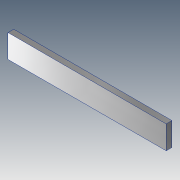
# Autodesk Inventor part: Y table support
Saved by Autodesk Inventor 2019 (Build 230136000, 136)
## iProperties
Created: 2018-10-20
Part Number: Y table support
Material: Aluminum 6061
Document SubType Name: Modeling
Designer: LillaHunden
Density: 2.7 g/cm^3
Appearance: Aluminum - Flat
Mass: 304.022 g
Surface Area: 289.886 cm^2
Volume: 112.601 cm^3
Author: LillaHunden
Autodesk Inventor part; units mm, degrees
ref_plane "YZ Plane" through (0, 0, 0) normal (1, 0, 0) x (0, 1, 0)
ref_plane "XZ Plane" through (0, 0, 0) normal (0, 1, 0) x (-1, 0, 0)
ref_plane "XY Plane" through (0, 0, 0) normal (0, 0, 1) x (1, 0, 0)
sketch "Sketch1" plane through (0, 0, 0) normal (0, 0, 1) x (1, 0, 0)
  line L0 (222.4, 4.1007) -> (192.16, 4.1007) construction
  line L1 (-50, 0) -> (232, 0) construction
  line L2 (232, 0) -> (232, 8) construction
  line L3 (-50, 8) -> (232, 8) construction
  line L4 (-50, 0) -> (-50, 8) construction
  line L5 (232, 0) -> (-50, 0)
  line L6 (-50, 0) -> (-50, 40)
  line L7 (-50, 40) -> (232, 40)
  line L8 (232, 40) -> (232, 0)
  line L9 (-50, 0) -> (-50, 8)
  dimension "d1" = 40
  constraints: 20 end point, 2 parallel, 1 horizontal, 1 perpendicular
  measures "d1" distance of L5.end L6.end
extrude "Extrusion1" add sketch "Sketch1" along normal blind 9.9823
body "Solid1"
